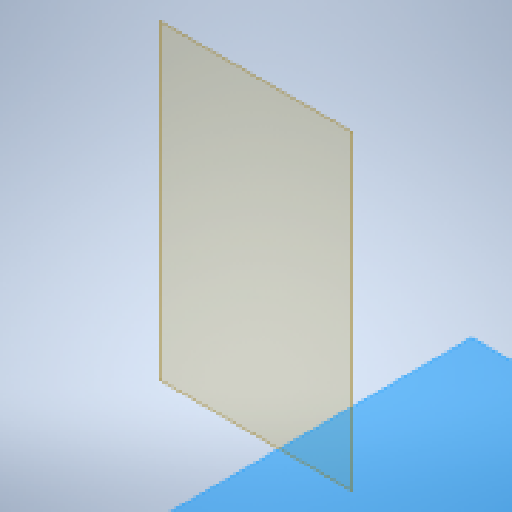
# Autodesk Inventor part: Union 4
Saved by Autodesk Inventor 2023 (Build 270158000, 158)
## iProperties
Created: 2023-05-14
Part Number: Union 4
Material: Genérico
Document SubType Name: Modeling
Designer: sergi
Density: 1 g/cm^3
Appearance: Valor por defecto
Author: sergi
Autodesk Inventor part; units mm, degrees
ref_plane "YZ Plane" through (0, 0, 0) normal (1, 0, 0) x (0, 1, 0)
ref_plane "XZ Plane" through (0, 0, 0) normal (0, 1, 0) x (-1, 0, 0)
ref_plane "XY Plane" through (0, 0, 0) normal (0, 0, 1) x (1, 0, 0)
ref_plane "Plano de trabajo5" through (0, 0, 0) normal (0, 0, 1) x (1, 0, 0)
sketch "Boceto2" plane through (0, 0, 0) normal (0, 0, 1) x (1, 0, 0)
  line L0 (0, 0) -> (20, 0)
  line L1 (20, 0) -> (20, -20)
  line L2 (20, -20) -> (0, -20)
  line L3 (0, -20) -> (0, 0)
  line L4 (0, -20) -> (6, -20)
  line L5 (6, -20) -> (6, -15)
  line L6 (6, -15) -> (6, -5)
  circle A0 centre (6, -15) radius 1.5
  circle A1 centre (6, -5) radius 1.5
  line L7 (20, -20) -> (20, -15)
  line L8 (20, -15) -> (16, -15)
  line L9 (16, -15) -> (16, -5)
  circle A2 centre (16, -15) radius 1.5
  circle A3 centre (16, -5) radius 1.5
  dimension "d17" = 20
  dimension "d18" = 20
  dimension "d19" = 6
  dimension "d20" = 5
  dimension "d21" = 10
  dimension "d22" = 3
  dimension "d23" = 3
  dimension "d24" = 5
  dimension "d25" = 4
  dimension "d26" = 10
  dimension "d27" = 3
  dimension "d28" = 3
  constraints: 20 end point, 4 centre point, 4 coincident, 4 perpendicular, 3 point on line, 2 parallel, 1 horizontal
  measures "d17" distance of L1.end L2.end
  measures "d18" distance of L0.end L1.end
  measures "d19" distance of L2.end L4.end
  measures "d20" distance of L4.end L5.end
  measures "d21" distance of L5.end L6.end
  measures "d22" diameter of A0
  measures "d23" diameter of A1
  measures "d24" distance of L1.end L7.end
  measures "d25" distance of L7.end L8.end
  measures "d26" distance of L8.end L9.end
  measures "d27" diameter of A2
  measures "d28" diameter of A3
extrude "Extrusión2" add sketch "Boceto2" along normal blind 3
fillet "Empalme2" radius 2 4 edges at (0, -20, 1.5) (0, 0, 1.5) (20, 0, 1.5) (20, -20, 1.5)
